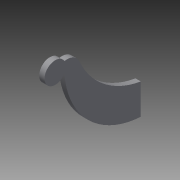
# Autodesk Inventor part: leg
Saved by Autodesk Inventor 2015 (Build 190159000, 159)
## iProperties
Created: 2015-06-21
Part Number: leg
Material: Generic
Document SubType Name: Modeling
Designer: Vu
Density: 1 g/cm^3
Appearance: Default
Author: Vu
Autodesk Inventor part; units mm, degrees
ref_plane "YZ Plane" through (0, 0, 0) normal (1, 0, 0) x (0, 1, 0)
ref_plane "XZ Plane" through (0, 0, 0) normal (0, 1, 0) x (-1, 0, 0)
ref_plane "XY Plane" through (0, 0, 0) normal (0, 0, 1) x (1, 0, 0)
sketch "Sketch1" plane through (0, 0, 0) normal (1, 0, 0) x (0, 1, 0)
  line L0 (0, 0) -> (0, -20)
  line L1 (0, 0) -> (20, 0) construction
  arc A0 (-50, 29.5654) -> (0, -20) centre (3.0398, 33.0683) ccw
  arc A1 (-40.1726, 31.4151) -> (0, 0) centre (8.9221, 52.8024) ccw
  arc A2 (-40.1726, 31.4151) -> (-50.0004, 36.5654) centre (-48.2889, 27.8794) ccw
  arc A3 (-50.0004, 36.5654) -> (-50, 29.5654) centre (-56.0624, 33.0651) ccw
  dimension "d0" = 20
  dimension "d1" = 90
  dimension "d2" = 50
  dimension "d3" = 10
  dimension "d5" = 7
  dimension "d6" = 7
  constraints: 9 point on circle, 4 centre point, 4 end point, 1 horizontal, 1 perpendicular, 1 tangent, 1 vertical
  measures "d0" distance of L0.start L0.end
  measures "d1" angle of L0 L1
  measures "d2" horizontal distance of L0.end A0.start
  measures "d3" distance of A0.start A1.start
  measures "d5" distance of A0.start A2.end
  measures "d6" radius of A3
extrude "Extrusion1" add sketch "Sketch1" along normal blind 3.5
body "Solid1"
